Autodesk Fusion 360 part; units mm, degrees
(part 2 of 2)
extrude "Extrude44" add sketch "Sketch18" along normal blind 9 separate body contours L0 L1 L2 L3 | A0 | A1 makes body 27
extrude "Extrude45" add sketch "Sketch18" against normal blind 5 contours A0 bodies 27
sketch "Sketch19" plane through (0, -5, 0) normal (0, -1, 0) x (1, 0, 0)
  circle A0 centre (95, 16) radius 4
  circle A1 centre (95, 16) radius 5
  constraint concentric A0 A1
extrude "Extrude46" add sketch "Sketch19" along normal blind 3 separate body makes body 28
sketch "Sketch20" plane through (0, 9, 0) normal (0, 1, 0) x (-1, 0, 0)
  line L0 (-85, 9) -> (-85, 23)
  line L1 (-85, 23) -> (-105, 23)
  line L2 (-105, 23) -> (-105, 9)
  line L3 (-105, 9) -> (-85, 9)
  line L4 (-85.2, 21) -> (-92.2, 21)
  line L5 (-92.2, 21) -> (-92.2, 13)
  line L6 (-92.2, 13) -> (-85.2, 13)
  line L7 (-85.2, 13) -> (-85.2, 21)
  line L8 (-97.5, 23) -> (-91.5, 23)
  line L9 (-91.5, 23) -> (-91.5, 28)
  line L10 (-91.5, 28) -> (-97.5, 28)
  line L11 (-97.5, 28) -> (-97.5, 23)
  line L12 (-95, 28) -> (-94, 28)
  line L13 (-94, 28) -> (-94, 38)
  line L14 (-94, 38) -> (-95, 38)
  line L15 (-95, 38) -> (-95, 28)
  line L16 (-94, 31) -> (-79, 31)
  line L17 (-94.5, 38) -> (-94.5, 28)
  line L18 (-94.5, 38) -> (-94.5, 46)
  spline S0 degree 5 poles (-94.5, 46) (-94.5062, 46.0548) (-94.4916, 46.1526) (-94.3888, 46.2635) (-94.0898, 46.3397) (-93.4601, 46.319) (-92.6306, 46.1979) (-91.6909, 46.001) (-90.7324, 45.7501) (-89.824, 45.4561) (-88.9828, 45.1082) (-88.1545, 44.667) (-87.2548, 44.0781) (-86.1965, 43.2834) (-84.9322, 42.2302) (-83.4688, 40.8893) (-81.9474, 39.2514) (-80.5351, 37.3914) (-79.3579, 35.4612) (-78.5272, 33.6503) (-78.1288, 32.1605) (-78.2076, 31.3717) (-78.5082, 31.0676) (-78.8179, 31) (-79, 31) knots 0 0 0 0 0 0 0.05 0.1 0.15 0.2 0.25 0.3 0.35 0.4 0.45 0.5 0.55 0.6 0.65 0.7 0.75 0.8 0.85 0.9 0.95 1 1 1 1 1 1
  line L19 (-78.1139, 31) -> (-79.8861, 31)
  line L20 (-86.2553, 43.5746) -> (-81.0569, 38.4579)
  line L21 (-93.5, 32) -> (-79.2324, 32)
  spline S1 degree 3 poles (-93.5, 45.298) (-93.434, 45.2916) (-93.365, 45.2838) (-93.2915, 45.2743) (-92.6221, 45.1885) (-91.6681, 44.978) (-90.8394, 44.7236) (-90.0681, 44.4868) (-89.43, 44.2284) (-88.7257, 43.8166) (-88.0442, 43.418) (-87.2395, 42.8442) (-86.1763, 41.952) (-85.0825, 41.0339) (-83.7164, 39.7678) (-82.4906, 38.2498) (-81.4355, 36.9432) (-80.4968, 35.4582) (-79.9111, 34.1902) (-79.5509, 33.4103) (-79.3268, 32.7101) (-79.258, 32.2578) (-79.2429, 32.1579) (-79.2348, 32.0705) (-79.2324, 32) knots 0.150463 0.150463 0.150463 0.150463 0.166325 0.166325 0.166325 0.310735 0.310735 0.310735 0.445145 0.445145 0.445145 0.575222 0.575222 0.575222 0.709058 0.709058 0.709058 0.82426 0.82426 0.82426 0.895113 0.895113 0.895113 0.910747 0.910747 0.910747 0.910747
  line L22 (-93.5, 38) -> (-93.5, 45.298)
  line L23 (-93.5, 38) -> (-93.5, 32)
  point P0 (-93.8066, 46.317)
  point P1 (-90, 45.5)
  point P2 (-83.6561, 41.0162)
  dimension "d328" = 7
  dimension "d329" = 8
  dimension "d330" = 2
  dimension "d331" = 0.2
  dimension "d334" = 15
  dimension "d335" = 8
  dimension "d336" = 1
  constraint horizontal L4
  constraint vertical L5
  constraint horizontal L6
  constraint vertical L7
  constraint horizontal L8
  constraint vertical L9
  constraint horizontal L10
  constraint vertical L11
  constraint coincident L1 L8.start
  constraint horizontal L12
  constraint vertical L13
  constraint horizontal L14
  constraint vertical L15
  constraint coincident L10 L12.start
  constraint coincident L13 L16.start
  constraint perpendicular L13 L16
  constraint midpoint L14 L17.start
  constraint midpoint L12 L17.end
  constraint perpendicular L14 L18
  constraint midpoint L16.end L19
  constraint coincident L16 L19.end
  constraint midpoint P2 L20
  measures "d328" distance of L4.start L4.end
  measures "d329" distance of L4.start L6.end
  measures "d330" distance of L1 L4
  measures "d331" distance of L0 L7
  measures "d334" distance of L16.start L16.end
  measures "d335" distance of L17.start L18.end
extrude "Extrude47" add sketch "Sketch20" along normal blind 3 contours L4 L5 L6 L7 bodies 27
extrude "Extrude48" add sketch "Sketch20" along normal blind 0.5 separate body contours L13 L14 L16 L18 S0 L19 makes body 29
pattern_circular "C-Pattern1" count 3 over 360 about axis through (94.5, 9, 38) along (0, 0, -1) of bodies 29 makes body 30 at (99.6602, 17.9378, 40.5351) makes body 31 at (99.6602, 0.0622, 40.5351)
extrude "Extrude49" add sketch "Sketch20" against normal blind 1 contours L1 L8 L9 L10 L11 L12 bodies 27
revolve "Revolve1" add sketch "Sketch20" angle 360 about axis through (94.5, 9, 38) along (0, 0, -1) contours L10 L12 L14 L15 L17 bodies 27 29 30 31
combine "Combine6" operation add target body 27 tool bodies 28
copy_body "Body->Comp9" bodies 27 removing the originals makes body 32 in component "Camera"
sketch "Sketch21" plane through (0, 0, 0) normal (0, 0, 1) x (1, 0, 0)
  line L0 (180, -80) -> (125, -80)
  line L1 (125, -80) -> (125, -43)
  line L2 (125, -43) -> (180, -43)
  line L3 (180, -43) -> (180, -80)
  dimension "d344" = 55
  dimension "d345" = 37
  constraint horizontal L0
  constraint vertical L1
  constraint horizontal L2
  constraint vertical L3
  measures "d344" distance of L0.start L0.end
  measures "d345" distance of L0.start L2.end
extrude "Extrude50" add sketch "Sketch21" along normal blind 7 separate body makes body 33
sketch "Sketch22" plane through (0, 0, 0) normal (0, 0, 1) x (1, 0, 0)
  line L0 (102.3222, 94.8297) -> (84.3222, 94.8297)
  line L1 (84.3222, 94.8297) -> (84.3222, 122.8297)
  line L2 (102.3222, 122.8297) -> (102.3222, 94.8297)
  line L3 (99.9222, 121.0297) -> (86.7222, 121.0297)
  line L4 (99.9222, 121.0297) -> (99.9222, 122.8297)
  line L5 (86.7222, 121.0297) -> (86.7222, 122.8297)
  line L6 (84.3222, 122.8297) -> (86.7222, 122.8297)
  line L7 (99.9222, 122.8297) -> (102.3222, 122.8297)
  line L8 (97.3222, 93.4297) -> (89.3222, 93.4297)
  line L9 (89.3222, 93.4297) -> (89.3222, 98.9297)
  line L10 (89.3222, 98.9297) -> (97.3222, 98.9297)
  line L11 (97.3222, 98.9297) -> (97.3222, 93.4297)
  dimension "d348" = 18
  dimension "d349" = 28
  dimension "d350" = 2.4
  dimension "d351" = 2.4
  dimension "d352" = 1.8
  dimension "d353" = 5
  dimension "d354" = 8
  dimension "d355" = 1.4
  dimension "d356" = 5.5
  constraint horizontal L0
  constraint vertical L1
  constraint horizontal L6
  constraint vertical L2
  constraint parallel L3 L6
  constraint coincident L4.end L6
  constraint perpendicular L4 L6
  constraint perpendicular L5 L6
  constraint collinear L6 L7
  constraint horizontal L8
  constraint vertical L9
  constraint horizontal L10
  constraint vertical L11
  measures "d348" distance of L0.start L0.end
  measures "d349" distance of L0.start L2.start
  measures "d350" distance of L1 L5
  measures "d351" distance of L2 L4
  measures "d352" distance of L3 L6
  measures "d353" distance of L1 L9
  measures "d354" distance of L9 L11
  measures "d355" distance of L0 L8
  measures "d356" distance of L8 L10
extrude "Extrude51" add sketch "Sketch22" against normal blind 1.7 separate body contours L0 L1 L2 L3 L4 L5 L6 L7 L9 L10 L11 | L0 L9 L10 L11 makes body 34
extrude "Extrude52" add sketch "Sketch22" along normal blind 3 contours L0 L8 L9 L11 | L0 L9 L10 L11 bodies 34
fillet "Fillet8" radius 1 2 edges at (97.3222, 96.1797, 3) (89.3222, 96.1797, 3) on bodies 34
chamfer "Chamfer4" distance 2 distance2 1.5 1 edges at (89.3222, 94.1297, 0) measured on face at (91.9889, 94.363, 0) on bodies 34
chamfer "Chamfer4" distance 2 distance2 1.5 1 edges at (97.3222, 94.1297, 0) measured on face at (91.9889, 94.363, 0) on bodies 34
copy_body "Body->Comp10" bodies 33 removing the originals makes body 35 in component "BattaryCam"
copy_body "Body->Comp11" bodies 34 removing the originals makes body 36 in component "ChargeModuleTP4056"
sketch "Sketch23" plane through (0, 0, 0) normal (0, 0, 1) x (1, 0, 0)
  line L0 (-135, -95) -> (-85, -95)
  line L1 (-85, -95) -> (-85, -155)
  line L2 (-85, -155) -> (-135, -155)
  line L3 (-135, -155) -> (-135, -95)
  circle A0 centre (-132, -98) radius 1.5
  circle A1 centre (-88, -98) radius 1.5
  circle A2 centre (-132, -152) radius 1.5
  circle A3 centre (-88, -152) radius 1.5
  line L4 (-129, -103) -> (-126.5, -103)
  line L5 (-126.5, -103) -> (-126.5, -142)
  line L6 (-126.5, -142) -> (-129, -142)
  line L7 (-129, -142) -> (-129, -103)
  line L8 (-111, -103) -> (-111, -142)
  line L9 (-113.5, -103) -> (-111, -103)
  line L10 (-113.5, -142) -> (-113.5, -103)
  line L11 (-111, -142) -> (-113.5, -142)
  line L12 (-106, -111) -> (-96, -111)
  line L13 (-96, -111) -> (-96, -131)
  line L14 (-96, -131) -> (-106, -131)
  line L15 (-106, -131) -> (-106, -111)
  dimension "d367" = 60
  dimension "d368" = 3
  dimension "d369" = 3
  dimension "d370" = 3
  dimension "d373" = 44
  dimension "d374" = -54
  dimension "d377" = 2.5
  dimension "d378" = 39
  dimension "d379" = 6
  dimension "d380" = 8
  dimension "d381" = 2.5
  dimension "d382" = 39
  dimension "d383" = 13
  dimension "d384" = 10
  dimension "d385" = 20
  dimension "d386" = 16
  dimension "d387" = 5
  constraint horizontal L0
  constraint vertical L1
  constraint horizontal L2
  constraint vertical L3
  constraint horizontal L4
  constraint vertical L5
  constraint horizontal L6
  constraint vertical L7
  constraint horizontal L9
  constraint vertical L8
  constraint horizontal L11
  constraint vertical L10
  constraint horizontal L12
  constraint vertical L13
  constraint horizontal L14
  constraint vertical L15
  measures "d367" distance of L0.start L2.end
  measures "d368" diameter of A0
  measures "d369" distance of L3 A0.centre
  measures "d370" distance of L0 A0.centre
  measures "d377" distance of L4.start L4.end
  measures "d378" distance of L4.start L6.end
  measures "d379" distance of L3 L7
  measures "d380" distance of L0 L4
  measures "d381" distance of L8.start L9.start
  measures "d382" distance of L10.start L9.start
  measures "d383" distance of L5 L10
  measures "d384" distance of L12.start L12.end
  measures "d385" distance of L12.start L14.end
  measures "d386" distance of L0 L12
  measures "d387" distance of L8 L15
extrude "Extrude53" add sketch "Sketch23" against normal blind 1.5 separate body contours L0 L1 L2 L3 | L4 L5 L6 L7 | L8 L9 L10 L11 | L12 L13 L14 L15 makes body 37
extrude "Extrude54" add sketch "Sketch23" along normal blind 9 contours L4 L5 L6 L7 | L8 L9 L10 L11 bodies 37
extrude "Extrude55" add sketch "Sketch23" along normal blind 8 contours L12 L13 L14 L15 bodies 37
copy_body "Body->Comp12" bodies 37 removing the originals makes body 38 in component "MainBoardCustom"
sketch "Sketch24" plane through (0, 0, 0) normal (0, 0, 1) x (1, 0, 0)
  line L0 (-150, 200) -> (-120, 200)
  line L1 (-120, 200) -> (-120, 165)
  line L2 (-120, 165) -> (-150, 165)
  line L3 (-150, 165) -> (-150, 200)
  circle A0 centre (-147, 197) radius 1.5
  circle A1 centre (-123, 197) radius 1.5
  circle A2 centre (-147, 168) radius 1.5
  circle A3 centre (-123, 168) radius 1.5
  line L4 (-143, 198) -> (-135.5, 198)
  line L5 (-135.5, 198) -> (-135.5, 192)
  line L6 (-135.5, 192) -> (-143, 192)
  line L7 (-143, 192) -> (-143, 198)
  line L8 (-126.5, 198) -> (-126.5, 192)
  line L9 (-134, 198) -> (-126.5, 198)
  line L10 (-134, 192) -> (-134, 198)
  line L11 (-126.5, 192) -> (-134, 192)
  line L12 (-127.2624, 184.2376) -> (-127.2624, 191.7376)
  line L13 (-127.2624, 191.7376) -> (-121.2624, 191.7376)
  line L14 (-121.2624, 191.7376) -> (-121.2624, 184.2376)
  line L15 (-121.2624, 184.2376) -> (-127.2624, 184.2376)
  line L16 (-121.2624, 183.7376) -> (-121.2624, 176.2376)
  line L17 (-127.2624, 183.7376) -> (-121.2624, 183.7376)
  line L18 (-127.2624, 176.2376) -> (-127.2624, 183.7376)
  line L19 (-121.2624, 176.2376) -> (-127.2624, 176.2376)
  line L20 (-129.3404, 175.6596) -> (-121.8404, 175.6596)
  line L21 (-121.8404, 175.6596) -> (-121.8404, 169.6596)
  line L22 (-121.8404, 169.6596) -> (-129.3404, 169.6596)
  line L23 (-129.3404, 169.6596) -> (-129.3404, 175.6596)
  line L24 (-143.3482, 190.6518) -> (-143.3482, 183.1518)
  line L25 (-149.3482, 190.6518) -> (-143.3482, 190.6518)
  line L26 (-149.3482, 183.1518) -> (-149.3482, 190.6518)
  line L27 (-143.3482, 183.1518) -> (-149.3482, 183.1518)
  dimension "d392" = 30
  dimension "d393" = 35
  dimension "d394" = 3
  dimension "d395" = 3
  dimension "d396" = 3
  dimension "d399" = 24
  dimension "d400" = -29
  dimension "d401" = 7.5
  dimension "d402" = 6
  dimension "d403" = 7
  dimension "d404" = 7.5
  dimension "d405" = 6
  dimension "d406" = 7.5
  dimension "d407" = 6
  dimension "d408" = 7.5
  dimension "d409" = 6
  dimension "d410" = 7.5
  dimension "d411" = 6
  dimension "d412" = 7.5
  dimension "d413" = 6
  constraint horizontal L0
  constraint vertical L1
  constraint horizontal L2
  constraint vertical L3
  constraint horizontal L4
  constraint vertical L5
  constraint horizontal L6
  constraint vertical L7
  constraint horizontal L9
  constraint vertical L8
  constraint horizontal L11
  constraint vertical L10
  measures "d392" distance of L0.start L0.end
  measures "d393" distance of L0.start L2.end
  measures "d394" diameter of A0
  measures "d395" distance of L0 A0.centre
  measures "d396" distance of L3 A0.centre
  measures "d401" distance of L5 L7
  measures "d402" distance of L4 L6
  measures "d403" distance of L3 L7
  measures "d404" distance of L8 L10
  measures "d405" distance of L9 L11
  measures "d406" distance of L13 L15
  measures "d407" distance of L12 L14
  measures "d408" distance of L17 L19
  measures "d409" distance of L16 L18
  measures "d410" distance of L21 L23
  measures "d411" distance of L20 L22
  measures "d412" distance of L25 L27
  measures "d413" distance of L24 L26
extrude "Extrude56" add sketch "Sketch24" against normal blind 1.5 separate body contours L0 L1 L2 L3 | L4 L5 L6 L7 | L8 L9 L10 L11 | L12 L13 L14 L15 | L16 L17 L18 L19 | L20 L21 L22 L23 | L24 L25 L26 L27 makes body 39
extrude "Extrude57" add sketch "Sketch24" along normal blind 8 contours L4 L5 L6 L7 | L8 L9 L10 L11 | L12 L13 L14 L15 | L16 L17 L18 L19 | L20 L21 L22 L23 | L24 L25 L26 L27 bodies 39
ref_plane "WorkPlane2" through (-139.25, 188, 4) normal (0, -1, 0) x (1, 0, 0)
sketch "Sketch25" plane through (0, 188, 0) normal (0, -1, 0) x (-1, 0, 0)
  circle A0 through (142.2658, -3.7767, -4) (136.2658, -0.3126, -4) (136.2658, -7.2408, -4)
  dimension "d419" = 8
extrude "Extrude58" add sketch "Sketch25" along normal blind 13 separate body contours A0 in plane through (0, 192, 0) normal (0, -1, 0) makes body 40
move_body "Move3" bodies 40 to x (1, 0, 0) y (0, 1, 0) z (0, 0, 1) at (0, -3.5, 0)
fillet "Fillet9" radius 1 1 edges at (-134.5365, 175.5, 5.2232) on bodies 40
fillet "Fillet10" radius 0.5 1 edges at (-134.5365, 188.5, 5.2232) on bodies 40
combine "Combine7" operation add target body 39 tool bodies 40
copy_body "Body->Comp13" bodies 39 removing the originals makes body 41 in component "CommutationBoard"
sketch "Sketch26" plane through (0, 0, 0) normal (0, 0, 1) x (1, 0, 0)
  line L0 (25, 195) -> (60, 195)
  line L1 (60, 195) -> (60, 170)
  line L2 (60, 170) -> (25, 170)
  line L3 (25, 170) -> (25, 195)
  circle A0 centre (28, 182.5) radius 1.25
  circle A1 centre (57, 182.5) radius 1.25
  line L4 (28, 182.5) -> (57, 182.5)
  dimension "d426" = 35
  dimension "d427" = 25
  dimension "d428" = 2.5
  dimension "d430" = 2.5
  dimension "d434" = 3
  dimension "d435" = 3
  constraint horizontal L0
  constraint vertical L1
  constraint horizontal L2
  constraint vertical L3
  constraint horizontal L4
  constraint symmetric L0 L2 L4
  constraint coincident A0.centre L4.start
  constraint coincident A1.centre L4.end
  measures "d426" distance of L0.start L0.end
  measures "d427" distance of L0.start L2.end
  measures "d428" diameter of A0
  measures "d430" diameter of A1
  measures "d434" distance of L3 A0.centre
  measures "d435" distance of L1 A1.centre
extrude "Extrude60" add sketch "Sketch26" along normal blind 1.5 separate body makes body 42
copy_body "Body->Comp15" bodies 42 removing the originals makes body 43 in component "FPVBoard"
component "MotorReductor" placed x (1, 0, 0) y (0, 1, 0) z (0, 0, 1) at (0, 0, 0)
component "Encoder" placed x (1, 0, 0) y (0, 1, 0) z (0, 0, 1) at (0, 0, 0)
component "BattaryHolder" placed x (1, 0, 0) y (0, 1, 0) z (0, 0, 1) at (0, 0, 0)
component "MaketNano" placed x (1, 0, 0) y (0, 1, 0) z (0, 0, 1) at (0, 0, 0)
component "MotorDriver" placed x (1, 0, 0) y (0, 1, 0) z (0, 0, 1) at (0, 0, 0)
component "MotorDriver2" placed x (1, 0, 0) y (0, 1, 0) z (0, 0, 1) at (0, 0, 0)
component "ChargeModule" placed x (1, 0, 0) y (0, 1, 0) z (0, 0, 1) at (0, 0, 0)
component "PowerSwitcher" placed x (1, 0, 0) y (0, 1, 0) z (0, 0, 1) at (0, 0, 0)
component "Camera" placed x (1, 0, 0) y (0, 1, 0) z (0, 0, 1) at (0, 0, 0)
component "BattaryCam" placed x (1, 0, 0) y (0, 1, 0) z (0, 0, 1) at (0, 0, 0)
component "ChargeModuleTP4056" placed x (1, 0, 0) y (0, 1, 0) z (0, 0, 1) at (0, 0, 0)
component "MainBoardCustom" placed x (1, 0, 0) y (0, 1, 0) z (0, 0, 1) at (0, 0, 0)
component "CommutationBoard" placed x (1, 0, 0) y (0, 1, 0) z (0, 0, 1) at (0, 0, 0)
component "FPVBoard" placed x (1, 0, 0) y (0, 1, 0) z (0, 0, 1) at (0, 0, 0)
equation "d261 = d260"
equation "d263 = d262"
